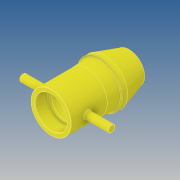
# Autodesk Inventor part: canon_support_entree
Saved by Autodesk Inventor 2019 (Build 230136000, 136)
## iProperties
Created: 2018-05-05
Part Number: canon_support_entree
Material: Générique
Document SubType Name: Modeling
Designer: Theo
Density: 1 g/cm^3
Appearance: Jaune canari
Author: Theo
Autodesk Inventor part; units mm, degrees
ref_plane "XZ Plane" through (0, 0, 0) normal (0, 1, 0) x (-1, 0, 0)
ref_plane "XY Plane" through (0, 0, 0) normal (0, 0, 1) x (1, 0, 0)
sketch "Esquisse1" plane through (0, 0, 0) normal (1, 0, 0) x (0, 1, 0)
  line L0 (0, 0) -> (0, -16.8642)
  line L1 (12.75, -0.5) -> (12.75, -10) construction
  line L2 (13, -0.5) -> (13, -10)
  line L3 (13.5, 0) -> (16.25, 0)
  line L4 (16.25, 0) -> (16.5, -0.25)
  line L5 (16.5, -0.25) -> (16.5, -29.75)
  line L6 (12.75, -64.25) -> (12.75, -12)
  line L7 (13, -10) -> (11.25, -10)
  line L8 (12.75, -12) -> (11.25, -12)
  line L9 (11.25, -10) -> (11.25, -12)
  line L10 (11, -10) -> (11, -12) construction
  line L11 (13.5, 0) -> (13, -0.5)
  line L12 (12.5, -12) -> (12.5, -64.25) construction
  line L13 (12.5, -0.5) -> (12.5, -10) construction
  line L14 (16.5, -29.75) -> (17.25, -39.75)
  line L15 (17.25, -39.75) -> (17.75, -40.25)
  line L16 (17.75, -40.25) -> (18.75, -40.25)
  line L17 (18.75, -40.25) -> (18.75, -44.25)
  line L18 (18.75, -44.25) -> (12.75, -64.25)
  dimension "d2" = 0.25
  dimension "d3" = 0.25
  dimension "d8" = 33
  dimension "d9" = 0.25
  dimension "d13" = 0.25
  dimension "d14" = 22
  dimension "d15" = 10
  dimension "d16" = 0.5
  dimension "d17" = 0.5
  dimension "d18" = 25
  dimension "d19" = 0.25
  dimension "d20" = 2
  dimension "d21" = 0.25
  dimension "d22" = 25
  dimension "d23" = 0.5
  dimension "d24" = 10
  dimension "d25" = 0.75
  dimension "d26" = 0.5
  dimension "d28" = 40.25
  dimension "d45" = 64.25
  dimension "d51" = 1
  dimension "d52" = 20
  dimension "d54" = 4
  constraints: 39 end point, 10 vertical, 9 horizontal alignment, 4 horizontal
  measures "d2" horizontal distance of L3.end L4.end
  measures "d3" horizontal distance of L3.end L4.end
  measures "d8" diameter of L5 L0
  measures "d9" distance between parallel lines of L2 L1
  measures "d13" distance between parallel lines of L9 L10
  measures "d14" diameter of L10 L0
  measures "d15" distance from line of L3.start L7
  measures "d16" horizontal distance of L3.start L2.start
  measures "d17" horizontal distance of L3.start L2.start
  measures "d18" diameter of L12 L0
  measures "d19" distance between parallel lines of L6 L12
  measures "d20" distance between parallel lines of L8 L7
  measures "d21" distance between parallel lines of L1 L13
  measures "d22" diameter of L13 L0
  measures "d23" horizontal distance of L14.end L15.end
  measures "d24" vertical distance of L5.end L14.end
  measures "d25" horizontal distance of L5.end L14.end
  measures "d26" horizontal distance of L14.end L15.end
  measures "d28" distance from line of L15.end L3
  measures "d45" vertical distance of L6.start L3.start
  measures "d51" distance from line of L15.end L17
  measures "d52" vertical distance of L17.end L6.start
  measures "d54" distance of L16.end L17.end
revolve "Révolution1" add sketch "Esquisse1" angle 360 about axis through (0, 0, 0) along (0, 0, -1)
ref_plane "Plan de construction1" through (16.5, 0, -15) normal (1, 0, 0) x (0, 1, 0)
sketch "Esquisse2" plane through (16.5, 0, -15) normal (1, 0, 0) x (0, 1, 0)
  circle A0 centre (0, 1.5) radius 3
  line L0 (0, -62.1) -> (0, 27.85) projected
  line L1 (-16.25, 15) -> (16.25, 15) projected
  point P0 (0, 15)
  dimension "d29" = 6
  dimension "d30" = 13.5
  constraints: 1 centre point, 1 point on line
  measures "d29" diameter of A0
  measures "d30" distance from line of A0.centre L1
extrude "Extrusion1" add sketch "Esquisse2" along normal blind 20 and the other way blind 0.5
chamfer "Chanfrein1" distance 0.5 angle 45 4 edges at (36.5, -3, -13.5) (16.3413, 2.2832, -11.554) (16.225, -3, -13.4926) (16.3418, 2.2797, -15.4502)
pattern_circular "Réseau circulaire1" count 2 over 360 about axis through (0, 0, -10) along (0, 0, 1) of "Extrusion1", "Chanfrein1"
equation "\"d3\" = d2"
equation "\"d17\" = d16"
